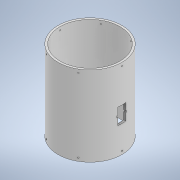
# Autodesk Inventor part: Aperture
Saved by Autodesk Inventor 2022 (Build 260153000, 153)
## iProperties
Created: 2023-08-20
Part Number: Aperture
Material: Generic
Document SubType Name: Modeling
Designer: fouad
Density: 1 g/cm^3
Appearance: Default
Author: fouad
Autodesk Inventor part; units mm, degrees
ref_plane "YZ Plane" through (0, 0, 0) normal (1, 0, 0) x (0, 1, 0)
ref_plane "XZ Plane" through (0, 0, 0) normal (0, 1, 0) x (-1, 0, 0)
ref_plane "XY Plane" through (0, 0, 0) normal (0, 0, 1) x (1, 0, 0)
sketch "Sketch1" plane through (0, 0, 0) normal (0, 1, 0) x (-1, 0, 0)
  circle A0 centre (0, 0) radius 18.735
  circle A1 centre (0, 0) radius 20
  dimension "d0" = 37.47
  dimension "d1" = 40
  constraints: 2 centre point, 2 coincident
  measures "d0" diameter of A0
  measures "d1" diameter of A1
extrude "Extrusion1" add sketch "Sketch1" along normal blind 50
ref_plane "Work Plane3" through (0, 21.88, 0) normal (0, -1, 0) x (1, 0, 0)
sketch "Sketch8" plane through (0, 21.88, 0) normal (0, -1, 0) x (1, 0, 0)
  line L0 (21.2099, 2.5) -> (18.2099, 2.5)
  line L1 (18.2099, 2.5) -> (18.2099, -2.5)
  line L2 (18.2099, -2.5) -> (21.2099, -2.5)
  line L3 (21.2099, -2.5) -> (21.2099, 2.5)
  circle A0 centre (0, 0) radius 18.735 projected
  line L4 (0, 0) -> (0, 8.02)
  line L5 (-21.2099, 2.5) -> (-18.2099, 2.5)
  line L6 (-18.2099, 2.5) -> (-18.2099, -2.5)
  line L7 (-18.2099, -2.5) -> (-21.2099, -2.5)
  line L8 (-21.2099, -2.5) -> (-21.2099, 2.5)
  dimension "d35" = 3
  dimension "d36" = 5
  dimension "d37" = 2.5
  constraints: 18 end point, 4 symmetric about line, 2 parallel, 1 horizontal, 1 perpendicular, 1 vertical
  measures "d35" distance of L2.end L1.end
  measures "d36" distance of L1.end L0.end
  measures "d37" distance from line of point (0, 0) L0
extrude "Extrusion9" cut sketch "Sketch8" along normal mid plane 10 contours L3 L2 A0 L0 | A0 L2 L1 L0 | L5 L6 L7 A0 | A0 L7 L8 L5
sketch "Sketch9" plane through (0, 21.88, 0) normal (0, -1, 0) x (1, 0, 0)
  line L0 (-21, 3) -> (-18, 3)
  line L1 (-18, 3) -> (-18, -3)
  line L2 (-18, -3) -> (-21, -3)
  line L3 (-21, -3) -> (-21, 3)
  circle A0 centre (0, 0) radius 20 projected
  circle A1 centre (0, 0) radius 18.735 projected
  line L4 (0, 0) -> (0, 5.4262)
  line L5 (21, 3) -> (18, 3)
  line L6 (18, 3) -> (18, -3)
  line L7 (18, -3) -> (21, -3)
  line L8 (21, -3) -> (21, 3)
  dimension "d42" = 3
  dimension "d43" = 6
  dimension "d44" = 3
  dimension "d46" = 18
  constraints: 18 end point, 4 symmetric about line, 2 parallel, 1 horizontal, 1 perpendicular, 1 vertical
  measures "d42" distance of L1.end L2.end
  measures "d43" distance of L0.end L1.end
  measures "d44" distance from line of point (0, 0) L0
  measures "d46" distance from line of L4.start L1
extrude "Extrusion10" cut sketch "Sketch9" along normal mid plane 1 contours L0 A0 L2 L3 | L0 A1 L2 A0 | L0 L1 L2 A1 | L5 L8 L7 A0 | A0 L7 A1 L5 | A1 L7 L6 L5
ref_plane "Work Plane4" through (19.8431, 0, 2.5) normal (0.9921567, 0, 0.125) x (0, 1, 0)
ref_plane "Work Plane5" through (19.8431, 0, -2.5) normal (0.9921567, 0, -0.125) x (0, 1, 0)
sketch "Sketch13" plane through (0, 0, 0) normal (1, 0, 0) x (0, 1, 0)
  circle A0 centre (48, 0) radius 0.375
  line L0 (50, -20) -> (50, 20) projected
  point P0 (0, 0)
  dimension "d64" = 0.75
  dimension "d70" = 2
  constraints: 1 centre point
  measures "d64" diameter of A0
  measures "d70" distance from line of L0 A0.centre
extrude "Extrusion13" cut sketch "Sketch13" against normal through all
pattern_circular "Circular Pattern1" count 6 over 360 about axis through (0, -10, 0) along (0, 1, 0) of "Extrusion13"
ref_plane "Work Plane6" through (0, 25, 0) normal (0, -1, 0) x (1, 0, 0)
mirror "Mirror2" about plane through (0, 25, 0) normal (0, -1, 0) of "Extrusion13", "Circular Pattern1"
body "Solid1"
